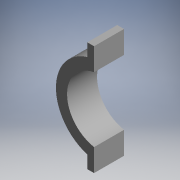
# Autodesk Inventor part: dremelClamp
Saved by Autodesk Inventor 2019 (Build 230136000, 136)
## iProperties
Created: 2019-05-13
Part Number: dremelClamp
Material: Generic
Document SubType Name: Modeling
Designer: Alex Jones
Density: 1 g/cm^3
Appearance: Default
Author: Alex Jones
Autodesk Inventor part; units mm, degrees
ref_plane "YZ Plane" through (0, 0, 0) normal (1, 0, 0) x (0, 1, 0)
ref_plane "XZ Plane" through (0, 0, 0) normal (0, 1, 0) x (-1, 0, 0)
ref_plane "XY Plane" through (0, 0, 0) normal (0, 0, 1) x (1, 0, 0)
sketch "Sketch1" plane through (0, 0, 0) normal (0, 0, 1) x (1, 0, 0)
  arc A0 (-11.3451, -36.1483) -> (17.6265, -10) centre (-17.6849, 0) ccw projected
  line L0 (17.6265, -10) -> (19.0151, -10) projected
  line L1 (19.0151, -10) -> (19.0151, 10) projected
  line L2 (19.0151, 10) -> (17.6265, 10) projected
  arc A1 (17.6265, 10) -> (-11.3451, 36.1483) centre (-17.6849, 0) ccw projected
  line L3 (-11.3451, 36.1483) -> (-11.3451, 46.225) projected
  line L4 (-17.6951, 46.225) -> (-11.3451, 46.225) projected
  line L5 (-17.6951, 25.4) -> (-17.6951, 46.225) projected
  arc A2 (-17.6951, -25.4) -> (-17.6951, 25.4) centre (-17.6849, 0) ccw projected
  line L6 (-17.6951, -46.225) -> (-17.6951, -25.4) projected
  line L7 (-17.6951, -46.225) -> (-11.3451, -46.225) projected
  line L8 (-11.3451, -36.1483) -> (-11.3451, -46.225) projected
  circle A3 centre (-17.6849, 0) radius 25.4
  arc A4 (-22.7296, 27.4808) -> (-22.7296, -27.4808) centre (-17.6849, 0) ccw
  line L9 (-22.7296, -46.5279) -> (-22.7296, -27.4808)
  line L10 (-22.7296, -46.5279) -> (-28.4927, -46.5279)
  line L11 (-22.7296, -27.4808) -> (-22.7296, 27.4808) construction
  arc A5 (-28.4927, 35.7486) -> (-28.4927, -35.7486) centre (-17.6849, 0) ccw
  line L12 (-22.7296, 27.4808) -> (-22.7296, 37.0044)
  line L13 (-28.4927, -46.5279) -> (-28.4927, -35.7486)
  line L14 (-17.6849, 0) -> (-81.3039, 0) construction
  line L15 (-22.7296, 46.5279) -> (-22.7296, 27.4808)
  line L16 (-22.7296, 46.5279) -> (-28.4927, 46.5279)
  line L17 (-28.4927, 46.5279) -> (-28.4927, 35.7486)
  point P0 (0, 0)
  dimension "d0" = 2.54
  dimension "d1" = 0
  dimension "d2" = 0.3029
  constraints: 18 end point, 4 point on circle, 3 centre point, 3 symmetric about line, 3 vertical, 2 coincident, 2 horizontal, 1 parallel
  measures "d0" radial gap between concentric circles of A3 A4
  measures "d1" radial gap between concentric circles of A2 A3
  measures "d2" distance between parallel lines of L7 L10
extrude "Extrusion1" add sketch "Sketch1" along normal blind 25.4 contours A4 L9 L10 L13 A5 L17 L16 L15 L12
sketch "Sketch2" plane through (-28.4927, 35.7486, 0) normal (-1, 0, 0) x (0, 0, 1)
  line L0 (0, -8.2678) -> (0, 10.7793) projected
  line L1 (25.4, 10.7793) -> (25.4, 0) projected
  line L2 (0, 10.7793) -> (25.4, 0) construction
  line L3 (12.7, 5.3897) -> (0, 5.3897) construction
  line L4 (12.7, 5.3897) -> (25.4, 5.3897) construction
  circle A0 centre (19.05, 5.3897) radius 3.175
  circle A1 centre (6.35, 5.3897) radius 3.175
  point P0 (0, -35.7486)
  dimension "d5" = 6.35
  constraints: 6 end point, 4 midpoint, 2 centre point, 1 equal radius, 1 perpendicular, 1 point on line
  measures "d5" diameter of A0
extrude "Extrusion2" cut sketch "Sketch2" against normal blind 25.4
ref_plane "Work Plane1" through (-28.4927, 0, 0) normal (0, 1, 0) x (1, 0, 0)
mirror "Mirror1" about plane through (-28.4927, 0, 0) normal (0, 1, 0) of "Extrusion2"
body "Solid1"
